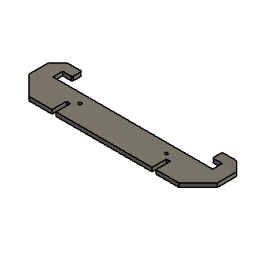
tablet_side_plate (Autodesk Fusion 360 design; units mm, degrees)
Autodesk Fusion 360 part; units mm, degrees
note: some values were not read from the file. Set by a fixed rule: the direction of a hole.
sketch "スケッチ1" plane through (0, 0, 0) normal (0, 1, 0) x (1, 0, 0)
  line L0 (98, 0) -> (98, 50)
  line L1 (98, 50) -> (73, 50)
  line L2 (73, 50) -> (73, 40)
  line L3 (73, 40) -> (83, 40)
  line L4 (83, 40) -> (83, 30)
  line L5 (83, 30) -> (-83, 30)
  line L6 (-83, 30) -> (-83, 40)
  line L7 (-83, 40) -> (-73, 40)
  line L8 (-73, 40) -> (-73, 50)
  line L9 (-73, 50) -> (-98, 50)
  line L10 (-98, 50) -> (-98, 0)
  line L11 (-98, 0) -> (-54, 0)
  line L12 (-54, 0) -> (-54, 15)
  line L13 (-54, 15) -> (-50, 15)
  line L14 (-50, 15) -> (-50, 0)
  line L15 (-50, 0) -> (50, 0)
  line L16 (50, 0) -> (50, 15)
  line L17 (50, 15) -> (54, 15)
  line L18 (54, 15) -> (54, 0)
  line L19 (54, 0) -> (98, 0)
  line L20 (-45, 20) -> (45, 20)
  point P0 (0, 30)
  dimension "d1" = 50
  dimension "d3" = 10
  dimension "d4" = 15
  dimension "d5" = 10
  dimension "d6" = 50
  dimension "d7" = 4
  dimension "d8" = 15
  dimension "d9" = 166
  dimension "d10" = 10
  dimension "d16" = 5
  dimension "d17" = 5
  dimension "d23" = 10
  constraint perpendicular L0 L1
  constraint perpendicular L1 L2
  constraint perpendicular L0 L3
  constraint perpendicular L1 L4
  constraint perpendicular L0 L5
  constraint perpendicular L1 L6
  constraint perpendicular L0 L7
  constraint perpendicular L1 L8
  constraint perpendicular L8 L9
  constraint perpendicular L1 L10
  constraint perpendicular L10 L11
  constraint perpendicular L11 L12
  constraint perpendicular L12 L13
  constraint perpendicular L13 L14
  constraint perpendicular L14 L15
  constraint perpendicular L15 L16
  constraint perpendicular L16 L17
  constraint perpendicular L17 L18
  constraint perpendicular L0 L19
  constraint midpoint origin L15
  constraint collinear L13 L17
  constraint equal L13 L17
  constraint collinear L15 L19
  constraint collinear L11 L15
  constraint midpoint L5 P0
  constraint vertical origin P0
  constraint vertical L0
  constraint equal L4 L6
  constraint equal L3 L7
  constraint collinear L1 L9
  constraint equal L1 L9
  constraint horizontal L20
  measures "d1" distance of L0.start L0.end
  measures "d3" distance of L3.end L4.end
  measures "d4" distance of L0 L4
  measures "d5" distance of L2 L4
  measures "d6" distance of origin L16
  measures "d7" distance of L16.end L17.end
  measures "d8" distance of L17.end L18.end
  measures "d9" distance of L4.end L5.end
  measures "d10" distance of L1.end L2.end
  measures "d16" distance of L14 L20.start
  measures "d17" distance of L16 L20.end
  measures "d23" distance of L5 L20
extrude "押し出し1" add sketch "スケッチ1" along normal blind 4
chamfer "面取り1" distance 20 angle 45 2 edges at (98, 2, 0) (-98, 2, 0)
chamfer "面取り2" distance 10 angle 45 2 edges at (98, 2, -50) (-98, 2, -50)
hole "穴1" at (45, 0, -20) at (-45, 0, -20) direction (0, 1, 0) diameter 3.2 depth 4 tip angle 118
fillet "フィレット1" radius 1 4 edges at (-73, 2, -40) (73, 2, -40) (73, 2, -50) (-73, 2, -50)
